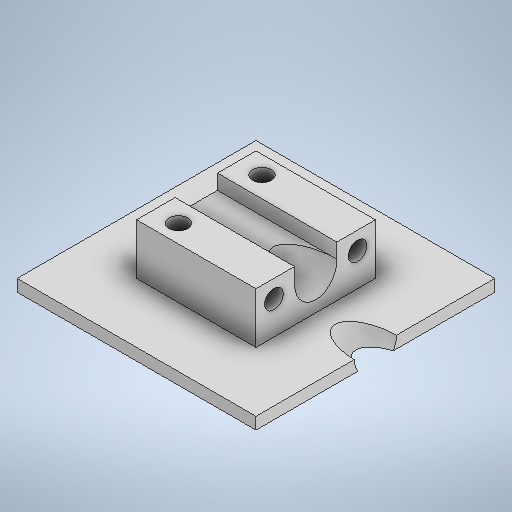
# Autodesk Inventor part: Camera Holder 1
Saved by Autodesk Inventor 2026.2 (Build 302298010, 298A)
## iProperties
Created: 2026-05-02
Part Number: Camera Holder 1
Material: Generic
Document SubType Name: Modeling
Designer: piete
Density: 1 g/cm^3
Appearance: Default
Author: piete
Autodesk Inventor part; units mm, degrees
ref_plane "YZ Plane" through (0, 0, 0) normal (1, 0, 0) x (0, 1, 0)
ref_plane "XZ Plane" through (0, 0, 0) normal (0, 1, 0) x (-1, 0, 0)
sketch "Sketch1" plane through (0, 0, 0) normal (0, 1, 0) x (-1, 0, 0)
  line L0 (20, 20) -> (-20, 20)
  line L1 (-20, 20) -> (-20, -20)
  line L2 (-20, -20) -> (20, -20)
  line L3 (20, -20) -> (20, 20)
  point P0 (0, 0)
  dimension "d0" = 40
  dimension "d1" = 40
  dimension "d2" = 20
  dimension "d3" = 20
  constraints: 8 end point, 2 parallel, 1 horizontal, 1 perpendicular
  measures "d0" distance of L1.end L2.end
  measures "d1" distance of L0.end L1.end
  measures "d2" distance from line of point (0, 0) L2
  measures "d3" distance from line of point (0, 0) L3
extrude "Extrusion1" add sketch "Sketch1" along normal blind 2
sketch "Sketch2" plane through (0, 2, 0) normal (0, 1, 0) x (1, 0, 0)
  line L0 (-10, -10) -> (10, -10)
  line L1 (10, -10) -> (10, 10)
  line L2 (10, 10) -> (-10, 10)
  line L3 (-10, 10) -> (-10, -10)
  point P0 (0, 0)
  dimension "d6" = 20
  dimension "d7" = 20
  dimension "d8" = 10
  dimension "d9" = 10
  constraints: 8 end point, 2 parallel, 1 horizontal, 1 perpendicular
  measures "d6" distance of L2.end L1.end
  measures "d7" distance of L1.end L0.end
  measures "d8" distance from line of L0 point (0, 0)
  measures "d9" distance from line of point (0, 0) L1
extrude "Extrusion2" add sketch "Sketch2" along normal blind 10
sketch "Sketch3" plane through (0, 12, 0) normal (0, 1, 0) x (1, 0, 0)
  line L0 (-10, 10) -> (-10, -10) projected
  line L1 (10, 10) -> (10, -10) projected
  line L2 (-10, -3.55) -> (10, -3.55)
  line L3 (10, -3.55) -> (10, 3.55)
  line L4 (10, 3.55) -> (-10, 3.55)
  line L5 (-10, 3.55) -> (-10, -3.55)
  point P0 (0, 0)
  point P1 (0, 3.55)
  point P2 (10, -3.55)
  dimension "d12" = 7.1
  dimension "d13" = 3.55
  constraints: 8 end point, 2 parallel, 2 point on line, 1 horizontal, 1 midpoint, 1 perpendicular
  measures "d12" distance of L3.end L2.end
  measures "d13" distance of point (0, 3.55) point (0, 0)
extrude "Extrusion3" cut sketch "Sketch3" against normal blind 4
ref_plane "Work Plane1" through (10, 8, 5) normal (0.866, -0.5, 0) x (0, 0, 1)
sketch "Sketch4" plane through (10, 8, 5) normal (0.866, -0.5, 0) x (0, 0, 1)
  line L0 (-1.45, 0) -> (-1.45, -3.4641) projected
  line L1 (-1.45, 10) -> (-8.55, 10) projected
  line L2 (-1.45, 0) -> (-1.45, 10) projected
  line L3 (-8.55, 0) -> (-1.45, 0) projected
  line L4 (-8.55, 10) -> (-8.55, 0) projected
  line L5 (-8.55, -3.4641) -> (-8.55, 0) projected
  circle A0 centre (-5, 0) radius 3.55
  point P0 (-5, 11.9282)
  constraints: 1 horizontal alignment, 1 midpoint, 2 other
extrude "Extrusion4" cut sketch "Sketch4" along normal through all both and the other way through all contours A0 L3 | L3 A0
sketch "Sketch5" plane through (0, 12, 0) normal (0, 1, 0) x (1, 0, 0)
  line L0 (10, -10) -> (-10, -10) projected
  line L1 (10, -3.55) -> (-10, -3.55) projected
  line L2 (-10, -10) -> (10, -10)
  line L3 (10, -10) -> (10, -3.55)
  line L4 (10, -3.55) -> (-10, -3.55)
  line L5 (-10, -3.55) -> (-10, -10)
  line L6 (-10, 3.0802) -> (10, 3.0802)
  line L7 (10, 3.0802) -> (10, 10.1436)
  line L8 (10, 10.1436) -> (-10, 10.1436)
  line L9 (-10, 10.1436) -> (-10, 3.0802)
  point P0 (0, 0)
  point P1 (-10, -3.55)
  constraints: 16 end point, 4 parallel, 2 horizontal, 2 perpendicular, 2 point on line
extrude "Extrusion5" cut sketch "Sketch5" against normal blind 1.5
sketch "Sketch6" plane through (0, 10.5, 0) normal (0, 1, 0) x (1, 0, 0)
  circle A0 centre (-6, -7) radius 1.55
  circle A1 centre (-6, 7) radius 1.55
  line L0 (-10, 3.55) -> (-10, 10) projected
  line L1 (-10, -10) -> (-10, -3.55) projected
  line L2 (10, -10) -> (-10, -10) projected
  line L3 (-10, 10) -> (10, 10) projected
  point P0 (0, 0)
  point P1 (-10, -6.775)
  point P2 (-10, 3.5772)
  dimension "d21" = 3.1
  dimension "d22" = 3.1
  dimension "d23" = 4
  dimension "d24" = 4
  dimension "d25" = 3
  dimension "d26" = 3
  constraints: 2 centre point, 1 midpoint
  measures "d21" diameter of A0
  measures "d22" diameter of A1
  measures "d23" distance from line of A1.centre L0
  measures "d24" horizontal distance of point (-10, -6.775) A0.centre
  measures "d25" distance from line of L2 A0.centre
  measures "d26" distance from line of L3 A1.centre
extrude "Extrusion6" cut sketch "Sketch6" against normal through all
sketch "Sketch7" plane through (10, 2, 10) normal (1, 0, 0) x (0, 0, -1)
  circle A0 centre (3, 5.5) radius 1.55
  circle A1 centre (17, 5.5) radius 1.55
  line L0 (20, 0) -> (20, 8.5) projected
  line L1 (0, 0) -> (0, 8.5) projected
  line L2 (6.45, 8.5) -> (0, 8.5) projected
  line L3 (20, 8.5) -> (13.55, 8.5) projected
  point P0 (10, -2)
  point P1 (13.5772, 8.7)
  dimension "d29" = 3.1
  dimension "d30" = 3.1
  dimension "d31" = 3
  dimension "d32" = 3
  dimension "d33" = 3
  dimension "d34" = 3
  constraints: 2 centre point, 1 other
  measures "d29" diameter of A0
  measures "d30" diameter of A1
  measures "d31" distance from line of L0 A1.centre
  measures "d32" distance from line of L1 A0.centre
  measures "d33" distance from line of L2 A0.centre
extrude "Extrusion7" cut sketch "Sketch7" against normal blind 10
equation "\"d2\" = 0.5 * d1"
equation "\"d3\" = 0.5 * d0"
equation "\"d8\" = 0.5 * d7"
equation "\"d9\" = 0.5 * d6"
equation "\"d13\" = 0.5 * d12"
body "Solid1"
